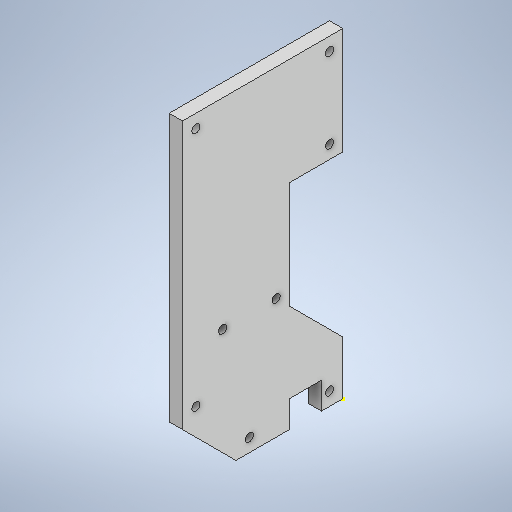
# Autodesk Inventor part: Lateral
Saved by Autodesk Inventor 2025.2 (Build 292293000, 293)
## iProperties
Created: 2025-01-27
Part Number: Lateral
Material: Genérico
Document SubType Name: Modeling
Designer: alex
Density: 1 g/cm^3
Appearance: Valor por defecto
Author: alex
Autodesk Inventor part; units mm, degrees
ref_plane "YZ Plane" through (0, 0, 0) normal (1, 0, 0) x (0, 1, 0)
ref_plane "XZ Plane" through (0, 0, 0) normal (0, 1, 0) x (-1, 0, 0)
ref_plane "XY Plane" through (0, 0, 0) normal (0, 0, 1) x (1, 0, 0)
sketch "Boceto1" plane through (0, 0, 0) normal (1, 0, 0) x (0, 1, 0)
  line L0 (0, 8) -> (10, 8)
  line L1 (10, 8) -> (10, 20)
  line L2 (10, 20) -> (0, 20)
  line L3 (20, 60) -> (0, 40)
  line L4 (0, 0) -> (20, 0)
  line L5 (40, 20) -> (20, 0)
  line L6 (20, 60) -> (40, 60)
  line L7 (0, 20) -> (0, 40)
  line L8 (0, 8) -> (0, 0)
  line L9 (40, 60) -> (120, 60)
  line L10 (120, 60) -> (120, 20)
  line L11 (80, 20) -> (80, 0)
  line L12 (80, 0) -> (120, 0)
  line L13 (120, 0) -> (120, 20)
  line L14 (40, 20) -> (80, 20)
  line L15 (120, 60) -> (115, 60)
  line L16 (120, 55) -> (120, 60)
  line L17 (20, 60) -> (25, 60)
  line L18 (120, 0) -> (115, 0)
  line L19 (120, 5) -> (120, 0)
  line L20 (0, 35) -> (0, 40)
  line L21 (0, 0) -> (5, 0)
  line L22 (0, 5) -> (0, 0)
  circle A0 centre (115, 55) radius 1.5
  circle A1 centre (115, 5) radius 1.5
  circle A2 centre (25, 55) radius 1.5
  circle A3 centre (5, 35) radius 1.5
  circle A4 centre (5, 5) radius 1.5
  line L23 (80, 0) -> (85, 0)
  line L24 (80, 5) -> (80, 0)
  circle A5 centre (85, 5) radius 1.5
  dimension "d2" = 8
  dimension "d3" = 10
  dimension "d4" = 12
  dimension "d5" = 40
  dimension "d7" = 20
  dimension "d11" = 20
  dimension "d12" = 20
  dimension "d13" = 20
  dimension "d16" = 100
  dimension "d17" = 60
  dimension "d18" = 40
  dimension "d27" = 3
  dimension "d28" = 3
  dimension "d29" = 3
  dimension "d30" = 3
  dimension "d31" = 3
  dimension "d34" = 3
  dimension "d35" = 5
  dimension "d36" = 5
  dimension "d37" = 5
  dimension "d38" = 5
  dimension "d39" = 5
  dimension "d40" = 5
  dimension "d41" = 5
  dimension "d42" = 5
  dimension "d43" = 5
  dimension "d44" = 5
  dimension "d45" = 5
  dimension "d46" = 5
  constraints: 50 end point, 9 horizontal, 6 centre point, 1 collinear, 1 parallel, 1 perpendicular, 1 vertical
  measures "d2" distance of L4.start L0.start
  measures "d3" distance of L0.start L0.end
  measures "d4" distance of L0.end L1.end
  measures "d5" distance of L4.start L3.end
  measures "d7" distance of L4.start L4.end
  measures "d11" distance from line of L4 L5.start
  measures "d12" distance of L2.end L3.end
  measures "d13" distance from line of L3.start L7
  measures "d16" distance from line of L3.start L10
  measures "d17" distance of L9.end L12.end
  measures "d18" distance of L11.end L12.end
  measures "d27" diameter of A0
  measures "d28" diameter of A1
  measures "d29" diameter of A2
  measures "d30" diameter of A3
  measures "d31" diameter of A4
  measures "d34" diameter of A5
  measures "d35" distance from line of L6 A2.centre
  measures "d36" horizontal distance of A2.centre L3.start
  measures "d37" distance from line of L15 A0.centre
  measures "d38" distance of L16.start A0.centre
  measures "d39" distance from line of L13 A1.centre
  measures "d40" distance from line of L12 A1.centre
  measures "d41" distance from line of L24 A5.centre
  measures "d42" distance from line of L12 A5.centre
  measures "d43" distance from line of L7 A3.centre
  measures "d44" horizontal distance of L3.end A3.centre
  measures "d45" distance from line of L8 A4.centre
  measures "d46" distance from line of L4 A4.centre
extrude "Extrusión1" add sketch "Boceto1" along normal blind 5
sketch "Boceto2" plane through (5, 0, 0) normal (1, 0, 0) x (0, 0, -1)
  point P0 (0, 0)
sketch "Boceto3" plane through (5, 0, 0) normal (1, 0, 0) x (0, 0, -1)
  circle A0 centre (-25, 45) radius 1.5
  line L0 (-20, 40) -> (-20, 80) projected
  circle A1 centre (-45, 45) radius 1.5
  point P0 (0, 0)
  dimension "d49" = 3
  dimension "d50" = 5
  dimension "d51" = 5
  dimension "d52" = 3
  dimension "d53" = 20
  dimension "d54" = 5
  constraints: 2 centre point
  measures "d49" diameter of A0
  measures "d50" distance from line of L0 A0.centre
  measures "d51" horizontal distance of L0.start A0.centre
  measures "d52" diameter of A1
  measures "d53" distance of A0.centre A1.centre
  measures "d54" vertical distance of L0.start A1.centre
extrude "Extrusión2" cut sketch "Boceto3" against normal blind 5
sketch "Boceto4" plane through (0, 0, 20) normal (0, -1, 0) x (1, 0, 0)
  point P0 (0, -20)
sketch "Boceto5" plane through (0, 0, 0) normal (0, -1, 0) x (1, 0, 0)
  circle A0 centre (2.5, 2.5) radius 1.5
  line L0 (0, 0) -> (5, 0) projected
  line L1 (0, 8) -> (0, 0) projected
  dimension "d57" = 3
  dimension "d58" = 2.5
  dimension "d59" = 2.5
  constraints: 1 centre point
  measures "d57" diameter of A0
  measures "d58" distance from line of L0 A0.centre
  measures "d59" distance from line of L1 A0.centre
extrude "Extrusión3" cut sketch "Boceto5" against normal blind 3
